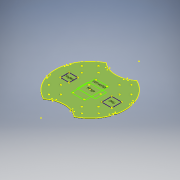
# Autodesk Inventor part: motherboard
Saved by Autodesk Inventor 2020 (Build 240168000, 168)
## iProperties
Created: 2024-11-03
Part Number: motherboard
Material: Медь
Document SubType Name: Modeling
Designer: Ivan
Density: 8.94 g/cm^3
Appearance: Оливково-зеленый
Mass: 442.829 g
Surface Area: 513.265 cm^2
Volume: 49.5335 cm^3
Author: Ivan
Autodesk Inventor part; units mm, degrees
ref_plane "YZ Plane" through (0, 0, 0) normal (1, 0, 0) x (0, 1, 0)
ref_plane "XZ Plane" through (0, 0, 0) normal (0, 1, 0) x (-1, 0, 0)
ref_plane "XY Plane" through (0, 0, 0) normal (0, 0, 1) x (1, 0, 0)
sketch "Эскиз2" plane through (0, 2, 127) normal (0, 1, 0) x (1, 0, 0)
  circle A0 centre (0, 127) radius 104
  line L0 (-92.1165, 78.7242) -> (-82.2877, 88.5529)
  line L1 (-82.2877, 88.5529) -> (-38.4471, 44.7123)
  line L2 (-38.4471, 44.7123) -> (-48.2758, 34.8835)
  line L3 (48.2758, 34.8835) -> (38.4471, 44.7123)
  line L4 (38.4471, 44.7123) -> (82.2877, 88.5529)
  line L5 (82.2877, 88.5529) -> (92.1165, 78.7242)
  line L6 (82.2877, 165.4471) -> (38.4471, 209.2877)
  line L7 (38.4471, 209.2877) -> (48.2758, 219.1165)
  line L8 (92.1165, 175.2758) -> (82.2877, 165.4471)
  line L9 (-48.2758, 219.1165) -> (-38.4471, 209.2877)
  line L10 (-38.4471, 209.2877) -> (-82.2877, 165.4471)
  line L11 (-82.2877, 165.4471) -> (-92.1165, 175.2758)
  point P0 (-84.409, 86.4316)
  point P1 (-80.1664, 86.4316)
  point P2 (-40.5684, 46.8336)
  point P3 (-40.5684, 42.591)
  point P4 (40.5684, 42.591)
  point P5 (40.5684, 46.8336)
  point P6 (80.1664, 86.4316)
  point P7 (84.409, 86.4316)
  point P8 (80.1664, 167.5684)
  point P9 (40.5684, 207.1664)
  point P10 (40.5684, 211.409)
  point P11 (84.409, 167.5684)
  point P12 (-40.5684, 211.409)
  point P13 (-40.5684, 207.1664)
  point P14 (-80.1664, 167.5684)
  point P15 (-84.409, 167.5684)
sketch "Эскиз3_1" plane through (0, 2, 127) normal (0, 1, 0) x (1, 0, 0)
  circle A0 centre (-23.8556, 50.0189) radius 1.5
  circle A1 centre (23.8556, 50.0189) radius 1.5
  circle A2 centre (-23.8556, 203.9811) radius 1.5
  circle A3 centre (23.8556, 203.9811) radius 1.5
  point P0 (0, 127)
sketch "Эскиз3" plane through (0, 0, 0) normal (0, 1, 0) x (-1, 0, 0)
  arc A0 (-36.9892, 97.1998) -> (36.9892, 97.1998) centre (0, 127) ccw projected
  line L0 (38.4471, 82.2877) -> (48.2758, 92.1165) projected
  line L1 (-48.2758, 92.1165) -> (-38.4471, 82.2877) projected
  arc A1 (-38.4471, 82.2877) -> (38.4471, 82.2877) centre (0, 133.1293) ccw
  circle A2 centre (0, 0) radius 69.3873 construction
  circle A3 centre (90.3481, 26.8924) radius 1.5 projected
  line L2 (82.2877, 38.4471) -> (38.4471, 82.2877) projected
  arc A4 (92.1165, -48.2758) -> (92.1165, 48.2758) centre (0, 0) ccw projected
  line L3 (104, 0) -> (-104.6293, 0) construction
  arc A5 (48.6356, -91.927) -> (-48.6356, -91.927) centre (0, -133.1293) ccw
  circle A6 centre (0, 0) radius 104
  arc A7 (38.4471, 82.2877) -> (48.5783, 91.8595) centre (0, 133.1293) ccw
  arc A8 (-48.6356, 91.927) -> (-38.4471, 82.2877) centre (0, 133.1293) ccw
  circle A9 centre (0, 0) radius 94.2655
  circle A10 centre (90.3481, -26.8924) radius 1.5 projected
  circle A11 centre (-90.3481, -26.8924) radius 1.5 projected
  circle A12 centre (-90.3481, 26.8924) radius 1.5 projected
  circle A13 centre (90.3481, 26.8924) radius 4
  circle A14 centre (90.3481, -26.8924) radius 4
  circle A15 centre (-90.3481, -26.8924) radius 4
  circle A16 centre (-90.3481, 26.8924) radius 4
  circle A17 centre (67.0849, 44.4575) radius 1.5 projected
  circle A18 centre (44.4575, 67.0849) radius 1.5 projected
  circle A19 centre (28.3991, 51.0265) radius 1.5 projected
  circle A20 centre (51.0265, 28.3991) radius 1.5 projected
  circle A21 centre (51.0265, -28.3991) radius 1.5 projected
  circle A22 centre (67.0849, -44.4575) radius 1.5 projected
  circle A23 centre (44.4575, -67.0849) radius 1.5 projected
  circle A24 centre (23.8556, 76.9811) radius 1.5 projected
  circle A25 centre (-23.8556, 76.9811) radius 1.5 projected
  circle A26 centre (23.8556, 76.9811) radius 4
  circle A27 centre (-23.8556, 76.9811) radius 4
  circle A28 centre (23.8556, -76.9811) radius 4
  circle A29 centre (-23.8556, -76.9811) radius 4
  point P0 (0, 69.3873)
  point P1 (60.3674, 60.3674)
  point P2 (38.4471, -82.2877)
  point P3 (-38.4471, -82.2877)
  point P4 (-41.4193, 84.6784)
  point P5 (-89.1259, 30.7011)
  point P6 (-91.4077, 23.0352)
  point P7 (-91.4077, -23.0352)
  point P8 (-89.1259, -30.7011)
  point P9 (-41.4193, -84.6784)
  point P10 (41.4193, -84.6784)
  point P11 (89.1259, -30.7011)
  point P12 (91.4077, -23.0352)
  point P13 (91.4077, 23.0352)
  point P14 (89.1259, 30.7011)
  point P15 (41.4193, 84.6784)
  point P16 (-27.6425, -75.6929)
  point P17 (-22.1541, -73.3611)
  point P18 (22.1541, -73.3611)
  point P19 (27.6425, -75.6929)
  point P20 (27.6425, 75.6929)
  point P21 (22.1541, 73.3611)
  point P22 (-22.1541, 73.3611)
  point P23 (-27.6425, 75.6929)
  dimension "d1" = 8
  constraints: 16 point on circle, 13 centre point, 10 coincident, 5 equal radius, 5 symmetric about line, 2 end point, 1 horizontal, 1 midpoint, 1 point on line, 1 vertical alignment, 7 other
  measures "d1" diameter of A13
extrude "Выдавливание1" add sketch "Эскиз3" along normal blind 2 contours A1 A27 A26 A7 A9 A13 A14 A5 A28 A29 A15 A16 A8
sketch "Эскиз1" plane through (0, 2, -127) normal (0, 1, 0) x (1, 0, 0)
  circle A0 centre (-90.3481, -100.1076) radius 1.5 projected
  circle A1 centre (90.3481, -153.8924) radius 1.5 projected
  circle A2 centre (-90.3481, -153.8924) radius 1.5 projected
  circle A3 centre (90.3481, -100.1076) radius 1.5 projected
  circle A4 centre (51.0265, -155.3991) radius 1.5 projected
  circle A5 centre (-67.0849, -171.4575) radius 1.5 projected
  circle A6 centre (-44.4575, -59.9151) radius 1.5 projected
  circle A7 centre (51.0265, -98.6009) radius 1.5 projected
  circle A8 centre (28.3991, -75.9735) radius 1.5 projected
  circle A9 centre (-67.0849, -82.5425) radius 1.5 projected
  circle A10 centre (-28.3991, -178.0265) radius 1.5 projected
  circle A11 centre (28.3991, -178.0265) radius 1.5 projected
  circle A12 centre (67.0849, -171.4575) radius 1.5 projected
  circle A13 centre (-51.0265, -155.3991) radius 1.5 projected
  circle A14 centre (-28.3991, -75.9735) radius 1.5 projected
  circle A15 centre (67.0849, -82.5425) radius 1.5 projected
  circle A16 centre (44.4575, -59.9151) radius 1.5 projected
  circle A17 centre (-51.0265, -98.6009) radius 1.5 projected
  circle A18 centre (-44.4575, -194.0849) radius 1.5 projected
  circle A19 centre (44.4575, -194.0849) radius 1.5 projected
  arc A20 (-36.9892, -29.8002) -> (36.9892, -29.8002) centre (0, 0) ccw projected
  arc A21 (-36.9892, -29.8002) -> (-48.2758, -34.8835) centre (0, -127) ccw projected
  line L0 (-48.2758, -34.8835) -> (-38.4471, -44.7123) projected
  line L1 (-38.4471, -44.7123) -> (-82.2877, -88.5529) projected
  line L2 (-82.2877, -88.5529) -> (-92.1165, -78.7242) projected
  arc A22 (-92.1165, -78.7242) -> (-92.1165, -175.2758) centre (0, -127) ccw projected
  line L3 (-92.1165, -175.2758) -> (-82.2877, -165.4471) projected
  line L4 (-82.2877, -165.4471) -> (-38.4471, -209.2877) projected
  line L5 (-38.4471, -209.2877) -> (-48.2758, -219.1165) projected
  arc A23 (-48.2758, -219.1165) -> (-36.9892, -224.1998) centre (0, -127) ccw projected
  arc A24 (36.9892, -224.1998) -> (-36.9892, -224.1998) centre (0, -254) ccw projected
  arc A25 (36.9892, -224.1998) -> (48.2758, -219.1165) centre (0, -127) ccw projected
  line L6 (48.2758, -219.1165) -> (38.4471, -209.2877) projected
  line L7 (38.4471, -209.2877) -> (82.2877, -165.4471) projected
  line L8 (82.2877, -165.4471) -> (92.1165, -175.2758) projected
  arc A26 (92.1165, -175.2758) -> (92.1165, -78.7242) centre (0, -127) ccw projected
  line L9 (92.1165, -78.7242) -> (82.2877, -88.5529) projected
  line L10 (82.2877, -88.5529) -> (38.4471, -44.7123) projected
  line L11 (38.4471, -44.7123) -> (48.2758, -34.8835) projected
  arc A27 (48.2758, -34.8835) -> (36.9892, -29.8002) centre (0, -127) ccw projected
  line L12 (-67.0849, -82.5425) -> (-51.0265, -98.6009) construction
  circle A28 centre (0, -127) radius 69.3873 projected
  line L13 (-62.0891, -96.0236) -> (-51.0265, -107.0862) projected
  line L14 (-51.0265, -107.0862) -> (-19.9138, -75.9735) projected
  line L15 (-19.9138, -75.9735) -> (-30.9764, -64.9109) projected
  line L16 (-51.0265, -146.9138) -> (-62.0891, -157.9764) projected
  line L17 (-19.9138, -178.0265) -> (-51.0265, -146.9138) projected
  line L18 (-30.9764, -189.0891) -> (-19.9138, -178.0265) projected
  line L19 (19.9138, -178.0265) -> (30.9764, -189.0891) projected
  line L20 (51.0265, -146.9138) -> (19.9138, -178.0265) projected
  line L21 (62.0891, -157.9764) -> (51.0265, -146.9138) projected
  line L22 (51.0265, -107.0862) -> (62.0891, -96.0236) projected
  line L23 (19.9138, -75.9735) -> (51.0265, -107.0862) projected
  line L24 (30.9764, -64.9109) -> (19.9138, -75.9735) projected
  point P0 (-59.0557, -90.5717)
  constraints: 1 other
hole "Отверстие1" at (-44.4575, 2, -67.0849) at (-67.0849, 2, -44.4575) at (-28.3991, 2, -51.0265) at (-51.0265, 2, -28.3991) at (44.4575, 2, -67.0849) at (67.0849, 2, -44.4575) at (28.3991, 2, -51.0265) at (51.0265, 2, -28.3991) at (51.0265, 2, 28.3991) at (67.0849, 2, 44.4575) at (44.4575, 2, 67.0849) at (28.3991, 2, 51.0265) at (-51.0265, 2, 28.3991) at (-28.3991, 2, 51.0265) at (-44.4575, 2, 67.0849) at (-67.0849, 2, 44.4575) direction (0, -1, 0) diameter 3 end through all
fillet "Сопряжение1" radius 4 16 edges at (-89.1259, 1, -30.7011) (-91.4077, 1, -23.0352) (-91.4077, 1, 23.0352) (-89.1259, 1, 30.7011) (89.1259, 1, -30.7011) (91.4077, 1, -23.0352) (91.4077, 1, 23.0352) (89.1259, 1, 30.7011) (-27.6425, 1, 75.6929) (-22.1541, 1, 73.3611) (27.6425, 1, 75.6929) (22.1541, 1, 73.3611) (-22.1541, 1, -73.3611) (-27.6425, 1, -75.6929) (27.6425, 1, -75.6929) (22.1541, 1, -73.3611)
sketch "Эскиз5" plane through (0, 2, 0) normal (0, 1, 0) x (1, 0, 0)
  line L0 (-15.1, 31) -> (15.1, 31) construction
  line L1 (15.1, 31) -> (15.1, -31) construction
  line L2 (15.1, -31) -> (-15.1, -31) construction
  line L3 (-15.1, -31) -> (-15.1, 31) construction
  line L4 (-15.1, 31) -> (15.1, -31) construction
  circle A0 centre (0, 0) radius 69.3873 projected
  arc A1 (92.1165, -48.2758) -> (92.1165, 48.2758) centre (0, 0) ccw projected
  arc A2 (-92.1117, 20.0355) -> (-92.1117, -20.0355) centre (0, 0) ccw projected
  dimension "d12" = 62
  dimension "d13" = 30.2
  constraints: 10 end point, 6 coincident, 2 parallel, 1 horizontal, 1 midpoint, 1 perpendicular
  measures "d12" distance of L0.end L1.end
  measures "d13" distance of L0.start L0.end
hole "Отверстие2" at (-15.1, 2, -31) at (15.1, 2, -31) at (15.1, 2, 31) at (-15.1, 2, 31) direction (0, -1, 0) diameter 3 end through all
sketch "Эскиз7" plane through (0, 2, 0) normal (0, 1, 0) x (1, 0, 0)
  line L0 (24.536, 3.71) -> (-12.5, 3.71)
  line L1 (-12.5, 3.71) -> (-12.5, 10)
  line L2 (24.536, 3.71) -> (24.536, 0)
  line L3 (0, 0) -> (-94.2655, 0) construction
  arc A0 (-92.1117, 20.0355) -> (-92.1117, -20.0355) centre (0, 0) ccw projected
  line L4 (0, 0) -> (0, -69.3873) construction
  arc A1 (20.9334, -72.9227) -> (-20.9334, -72.9227) centre (0, -133.1293) ccw projected
  circle A2 centre (24.536, 3.71) radius 1.5
  circle A3 centre (-12.5, 10) radius 1.5
  point P0 (0, 3.71)
  dimension "d21" = 37.036
  dimension "d22" = 6.29
  dimension "d23" = 3.71
  dimension "d24" = 24.536
  dimension "d25" = 3
  dimension "d26" = 3
  constraints: 10 end point, 3 point on line, 2 centre point, 2 coincident, 2 perpendicular, 2 point on circle, 1 horizontal, 1 parallel, 1 vertical
  measures "d21" distance from line of L1 L0.start
  measures "d22" distance from line of L0 L1.end
  measures "d23" distance from line of L0 L2.end
  measures "d24" distance from line of L2 point (0, 3.71)
  measures "d25" diameter of A2
  measures "d26" diameter of A3
extrude "Выдавливание2" cut sketch "Эскиз7" against normal through all
sketch "Эскиз8" plane through (0, 2, 0) normal (0, 1, 0) x (1, 0, 0)
  line L0 (45, 13.5) -> (72, 13.5)
  line L1 (72, 13.5) -> (72, -13.5)
  line L2 (72, -13.5) -> (45, -13.5)
  line L3 (45, -13.5) -> (45, 13.5)
  line L4 (0, 0) -> (-94.2655, 0) construction
  point P0 (45, 0)
  dimension "d29" = 27
  dimension "d30" = 45
  constraints: 8 end point, 4 coincident, 2 parallel, 2 perpendicular, 1 horizontal, 1 midpoint, 1 point on line
  measures "d29" distance of L0.start L0.end
  measures "d30" distance from line of L3 point (0, 0)
hole "Отверстие3" at (45, 2, -13.5) at (72, 2, -13.5) at (72, 2, 13.5) at (45, 2, 13.5) direction (0, -1, 0) diameter 3 end through all
sketch "Эскиз9" plane through (0, 2, 0) normal (0, 1, 0) x (1, 0, 0)
  line L0 (-68.8, 11.75) -> (-45, 11.75)
  line L1 (-45, 11.75) -> (-45, -11.75)
  line L2 (-45, -11.75) -> (-68.8, -11.75)
  line L3 (-68.8, -11.75) -> (-68.8, 11.75)
  line L4 (0, 0) -> (-94.2655, 0) construction
  line L5 (-45, 0) -> (-68.8, 0) construction
  point P0 (-56.9, 0)
  dimension "d38" = 23.5
  dimension "d39" = 23.8
  dimension "d49" = 45
  constraints: 10 end point, 3 midpoint, 3 perpendicular, 1 collinear
  measures "d38" distance from line of L2 L0.end
  measures "d39" distance from line of L3 L1.end
  measures "d49" distance from line of L1 point (0, 0)
hole "Отверстие4" at (-68.8, 2, -11.75) at (-45, 2, -11.75) at (-45, 2, 11.75) at (-68.8, 2, 11.75) direction (0, -1, 0) diameter 3 end through all
sketch "Эскиз10" plane through (0, 2, 0) normal (0, 1, 0) x (1, 0, 0)
  circle A0 centre (-45, -11.75) radius 1.5 projected
  circle A1 centre (-68.8, 11.75) radius 1.5 projected
  circle A2 centre (-45, 11.75) radius 1.5 projected
  circle A3 centre (-68.8, -11.75) radius 1.5 projected
  circle A4 centre (72, -13.5) radius 1.5 projected
  circle A5 centre (45, 13.5) radius 1.5 projected
  circle A6 centre (72, 13.5) radius 1.5 projected
  circle A7 centre (45, -13.5) radius 1.5 projected
  circle A8 centre (24.536, 3.71) radius 1.5 projected
  circle A9 centre (-12.5, 10) radius 1.5 projected
  circle A10 centre (15.1, -31) radius 1.5 projected
  circle A11 centre (-15.1, 31) radius 1.5 projected
  circle A12 centre (15.1, 31) radius 1.5 projected
  circle A13 centre (-15.1, -31) radius 1.5 projected
  arc A14 (23.0513, 73.0628) -> (20.9334, 72.9227) centre (22.2471, 69.1445) ccw projected
  arc A15 (-20.9334, 72.9227) -> (20.9334, 72.9227) centre (0, 133.1293) ccw projected
  arc A16 (-20.9334, 72.9227) -> (-23.0513, 73.0628) centre (-22.2471, 69.1445) ccw projected
  arc A17 (-27.2343, 74.8401) -> (-23.0513, 73.0628) centre (-23.8556, 76.9811) ccw projected
  arc A18 (-27.2343, 74.8401) -> (-28.8054, 76.2672) centre (-30.613, 72.699) ccw projected
  arc A19 (-41.4193, 84.6784) -> (-28.8054, 76.2672) centre (0, 133.1293) ccw projected
  arc A20 (-41.4193, 84.6784) -> (-88.0749, 33.5976) centre (0, 0) ccw projected
  arc A21 (-88.0749, 33.5976) -> (-87.3429, 29.5321) centre (-84.3376, 32.1719) ccw projected
  arc A22 (-89.2756, 23.0388) -> (-87.3429, 29.5321) centre (-90.3481, 26.8924) ccw projected
  arc A23 (-89.2756, 23.0388) -> (-92.1117, 20.0355) centre (-88.2031, 19.1853) ccw projected
  arc A24 (-92.1117, 20.0355) -> (-92.1117, -20.0355) centre (0, 0) ccw projected
  arc A25 (-92.1117, -20.0355) -> (-89.2756, -23.0388) centre (-88.2031, -19.1853) ccw projected
  arc A26 (-87.3429, -29.5321) -> (-89.2756, -23.0388) centre (-90.3481, -26.8924) ccw projected
  arc A27 (-87.3429, -29.5321) -> (-88.0749, -33.5976) centre (-84.3376, -32.1719) ccw projected
  arc A28 (-88.0749, -33.5976) -> (-41.4193, -84.6784) centre (0, 0) ccw projected
  arc A29 (-28.8054, -76.2672) -> (-41.4193, -84.6784) centre (0, -133.1293) ccw projected
  arc A30 (-28.8054, -76.2672) -> (-27.2343, -74.8401) centre (-30.613, -72.699) ccw projected
  arc A31 (-23.0513, -73.0628) -> (-27.2343, -74.8401) centre (-23.8556, -76.9811) ccw projected
  arc A32 (-23.0513, -73.0628) -> (-20.9334, -72.9227) centre (-22.2471, -69.1445) ccw projected
  arc A33 (20.9334, -72.9227) -> (-20.9334, -72.9227) centre (0, -133.1293) ccw projected
  arc A34 (20.9334, -72.9227) -> (23.0513, -73.0628) centre (22.2471, -69.1445) ccw projected
  arc A35 (27.2343, -74.8401) -> (23.0513, -73.0628) centre (23.8556, -76.9811) ccw projected
  arc A36 (27.2343, -74.8401) -> (28.8054, -76.2672) centre (30.613, -72.699) ccw projected
  arc A37 (41.4193, -84.6784) -> (28.8054, -76.2672) centre (0, -133.1293) ccw projected
  arc A38 (41.4193, -84.6784) -> (88.0749, -33.5976) centre (0, 0) ccw projected
  arc A39 (88.0749, -33.5976) -> (87.3429, -29.5321) centre (84.3376, -32.1719) ccw projected
  arc A40 (89.2756, -23.0388) -> (87.3429, -29.5321) centre (90.3481, -26.8924) ccw projected
  arc A41 (89.2756, -23.0388) -> (92.1117, -20.0355) centre (88.2031, -19.1853) ccw projected
  arc A42 (92.1117, -20.0355) -> (92.1117, 20.0355) centre (0, 0) ccw projected
  arc A43 (92.1117, 20.0355) -> (89.2756, 23.0388) centre (88.2031, 19.1853) ccw projected
  arc A44 (87.3429, 29.5321) -> (89.2756, 23.0388) centre (90.3481, 26.8924) ccw projected
  arc A45 (87.3429, 29.5321) -> (88.0749, 33.5976) centre (84.3376, 32.1719) ccw projected
  arc A46 (88.0749, 33.5976) -> (41.4193, 84.6784) centre (0, 0) ccw projected
  arc A47 (28.8054, 76.2672) -> (41.4193, 84.6784) centre (0, 133.1293) ccw projected
  arc A48 (28.8054, 76.2672) -> (27.2343, 74.8401) centre (30.613, 72.699) ccw projected
  arc A49 (23.0513, 73.0628) -> (27.2343, 74.8401) centre (23.8556, 76.9811) ccw projected
  circle A50 centre (44.4575, -67.0849) radius 1.5 projected
  circle A51 centre (51.0265, -28.3991) radius 1.5 projected
  circle A52 centre (28.3991, 51.0265) radius 1.5 projected
  circle A53 centre (44.4575, 67.0849) radius 1.5 projected
  circle A54 centre (-28.3991, 51.0265) radius 1.5 projected
  circle A55 centre (67.0849, 44.4575) radius 1.5 projected
  circle A56 centre (51.0265, 28.3991) radius 1.5 projected
  circle A57 centre (67.0849, -44.4575) radius 1.5 projected
  circle A58 centre (28.3991, -51.0265) radius 1.5 projected
  circle A59 centre (-51.0265, -28.3991) radius 1.5 projected
  circle A60 centre (-44.4575, 67.0849) radius 1.5 projected
  circle A61 centre (-51.0265, 28.3991) radius 1.5 projected
  circle A62 centre (-67.0849, -44.4575) radius 1.5 projected
  circle A63 centre (-67.0849, 44.4575) radius 1.5 projected
  circle A64 centre (-44.4575, -67.0849) radius 1.5 projected
  circle A65 centre (-28.3991, -51.0265) radius 1.5 projected
  circle A66 centre (-68.8, 11.75) radius 1.5 projected
  circle A67 centre (-45, -11.75) radius 1.5 projected
  line L0 (-68.8, 11.75) -> (-45, 11.75)
  line L1 (-45, 11.75) -> (-45, -11.75)
  line L2 (-45, -11.75) -> (-68.8, -11.75)
  line L3 (-68.8, -11.75) -> (-68.8, 11.75)
  circle A68 centre (45, 13.5) radius 1.5 projected
  circle A69 centre (72, -13.5) radius 1.5 projected
  line L4 (45, 13.5) -> (72, 13.5)
  line L5 (72, 13.5) -> (72, -13.5)
  line L6 (72, -13.5) -> (45, -13.5)
  line L7 (45, -13.5) -> (45, 13.5)
  line L8 (51.1518, 4.0105) -> (66.5748, 4.0105) construction
  line L9 (66.5748, 4.0105) -> (66.5748, -7.8728) construction
  line L10 (66.5748, -7.8728) -> (51.1518, -7.8728) construction
  line L11 (51.1518, -7.8728) -> (51.1518, 4.0105) construction
  line L12 (-69.206, 3.9661) -> (-52.0382, 3.9661) construction
  line L13 (-52.0382, 3.9661) -> (-52.0382, -4.3919) construction
  line L14 (-52.0382, -4.3919) -> (-69.206, -4.3919) construction
  line L15 (-69.206, -4.3919) -> (-69.206, 3.9661) construction
  line L16 (-20.5665, 15.2259) -> (28.8081, 15.2259)
  line L17 (28.8081, 15.2259) -> (28.8081, -14.3223)
  line L18 (28.8081, -14.3223) -> (-20.5665, -14.3223)
  line L19 (-20.5665, -14.3223) -> (-20.5665, 15.2259)
  line L20 (-8.4409, 4.6438) -> (14.3742, 4.6438) construction
  line L21 (14.3742, 4.6438) -> (14.3742, -9.3616) construction
  line L22 (14.3742, -9.3616) -> (-8.4409, -9.3616) construction
  line L23 (-8.4409, -9.3616) -> (-8.4409, 4.6438) construction
  line L24 (-18.55, 32.1896) -> (18.0912, 32.1896)
  line L25 (18.0912, 32.1896) -> (18.0912, -32.2758)
  line L26 (18.0912, -32.2758) -> (-18.55, -32.2758)
  line L27 (-18.55, -32.2758) -> (-18.55, 32.1896)
  line L28 (-16.0926, 28.048) -> (-1.086, 28.048) construction
  line L29 (-1.086, 28.048) -> (-1.086, 19.8626) construction
  line L30 (-1.086, 19.8626) -> (-16.0926, 19.8626) construction
  line L31 (-16.0926, 19.8626) -> (-16.0926, 28.048) construction
  constraints: 32 end point, 8 parallel, 4 horizontal, 4 perpendicular, 8 other
equation "\"d26\" = d25"
equation "\"d31\" = d25"
equation "\"d42\" = d25"
